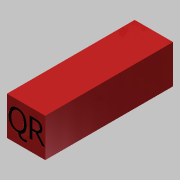
# Autodesk Inventor part: Container 2 2 5 colored color 4
Saved by Autodesk Inventor 2015 (Build 190159000, 159)
## iProperties
Created: 2015-03-07
Part Number: Container 2 2 5 colored color 4
Material: Generic
Document SubType Name: Modeling
Designer: Vukica
Density: 1 g/cm^3
Appearance: Light Red
Author: Vukica
Autodesk Inventor part; units mm, degrees
ref_plane "YZ Plane" through (0, 0, 0) normal (1, 0, 0) x (0, 1, 0)
ref_plane "XZ Plane" through (0, 0, 0) normal (0, 1, 0) x (-1, 0, 0)
ref_plane "XY Plane" through (0, 0, 0) normal (0, 0, 1) x (1, 0, 0)
sketch "Sketch1" plane through (0, 0, 0) normal (0, 0, 1) x (1, 0, 0)
  line L0 (0, 0) -> (38.1, 0)
  line L1 (38.1, 0) -> (38.1, 38.1)
  line L2 (38.1, 38.1) -> (0, 38.1)
  line L3 (0, 38.1) -> (0, 0)
  dimension "d0" = 38.1
  dimension "d1" = 38.1
  constraints: 8 end point, 2 parallel, 1 horizontal, 1 perpendicular
  measures "d0" distance of L1.end L2.end
  measures "d1" distance of L2.end L0.start
extrude "Extrusion1" add sketch "Sketch1" along normal blind 127
sketch "Sketch2" plane through (0, 0, 127) normal (0, 0, 1) x (1, 0, 0)
  line L0 (0.6292, 31.1418) -> (47.0243, 31.1418) construction
  line L1 (47.0243, 31.1418) -> (47.0243, -1.483) construction
  line L2 (47.0243, -1.483) -> (0.6292, -1.483) construction
  line L3 (0.6292, -1.483) -> (0.6292, 31.1418) construction
  spline S0 degree 2 poles (19.566, 5.4207) (18.825, 5.2396) (17.2112, 5.042) (16.4044, 5.042) knots 0 0 0 1 2 2 2
  spline S1 degree 2 poles (16.4044, 5.042) (14.1155, 5.042) (11.2667, 7.5944) (11.135, 9.9656) knots 0 0 0 1 2 2 2
  spline S2 degree 2 poles (11.135, 9.9656) (10.9539, 9.9656) (10.641, 9.9656) (10.5093, 9.9656) knots 0 0 0 1 2 2 2
  spline S3 degree 2 poles (10.5093, 9.9656) (8.4509, 9.9656) (5.1411, 11.3652) (3.9555, 12.732) knots 0 0 0 1 2 2 2
  spline S4 degree 2 poles (3.9555, 12.732) (2.7863, 14.0823) (1.5349, 18.0343) (1.5349, 20.5372) knots 0 0 0 1 2 2 2
  spline S5 degree 2 poles (1.5349, 20.5372) (1.5349, 23.1061) (2.8028, 26.9922) (3.972, 28.3754) knots 0 0 0 1 2 2 2
  spline S6 degree 2 poles (3.972, 28.3754) (5.1576, 29.7422) (8.4674, 31.1418) (10.5093, 31.1418) knots 0 0 0 1 2 2 2
  spline S7 degree 2 poles (10.5093, 31.1418) (12.5841, 31.1418) (15.9104, 29.6928) (17.063, 28.3754) knots 0 0 0 1 2 2 2
  spline S8 degree 2 poles (17.063, 28.3754) (18.2157, 27.0416) (19.5001, 23.0731) (19.5001, 20.5372) knots 0 0 0 1 2 2 2
  spline S9 degree 2 poles (19.5001, 20.5372) (19.5001, 16.5852) (16.4208, 11.4476) (13.7368, 10.5419) knots 0 0 0 1 2 2 2
  spline S10 degree 2 poles (13.7368, 10.5419) (13.8026, 9.7844) (14.1978, 8.5659) (14.5107, 8.2201) knots 0 0 0 1 2 2 2
  spline S11 degree 2 poles (14.5107, 8.2201) (14.8894, 7.792) (15.9268, 7.3968) (16.849, 7.3968) knots 0 0 0 1 2 2 2
  spline S12 degree 2 poles (16.849, 7.3968) (17.3924, 7.3968) (18.8744, 7.7426) (19.2037, 7.8743) knots 0 0 0 1 2 2 2
  line L4 (19.2037, 7.8743) -> (19.566, 7.8743)
  line L5 (19.566, 7.8743) -> (19.566, 5.4207)
  spline S13 degree 2 poles (16.6843, 20.5372) (16.6843, 22.5627) (15.8116, 25.6749) (15.0212, 26.6958) knots 0 0 0 1 2 2 2
  spline S14 degree 2 poles (15.0212, 26.6958) (14.2143, 27.7497) (11.9419, 28.8036) (10.5257, 28.8036) knots 0 0 0 1 2 2 2
  spline S15 degree 2 poles (10.5257, 28.8036) (9.0602, 28.8036) (6.8536, 27.7826) (6.0138, 26.6958) knots 0 0 0 1 2 2 2
  spline S16 degree 2 poles (6.0138, 26.6958) (5.207, 25.6584) (4.3507, 22.5133) (4.3507, 20.5372) knots 0 0 0 1 2 2 2
  spline S17 degree 2 poles (4.3507, 20.5372) (4.3507, 16.5358) (7.7099, 12.2709) (10.5257, 12.2709) knots 0 0 0 1 2 2 2
  spline S18 degree 2 poles (10.5257, 12.2709) (13.3416, 12.2709) (16.6843, 16.5358) (16.6843, 20.5372) knots 0 0 0 1 2 2 2
  line L6 (38.1899, 10.3937) -> (34.6825, 10.3937)
  line L7 (34.6825, 10.3937) -> (28.2605, 18.4789)
  line L8 (28.2605, 18.4789) -> (25.1647, 18.4789)
  line L9 (25.1647, 18.4789) -> (25.1647, 10.3937)
  line L10 (25.1647, 10.3937) -> (22.4641, 10.3937)
  line L11 (22.4641, 10.3937) -> (22.4641, 30.7137)
  line L12 (22.4641, 30.7137) -> (27.7006, 30.7137)
  spline S19 degree 2 poles (27.7006, 30.7137) (29.4461, 30.7137) (31.8008, 30.335) (32.8711, 29.6434) knots 0 0 0 1 2 2 2
  spline S20 degree 2 poles (32.8711, 29.6434) (33.9415, 28.9518) (35.1765, 26.7946) (35.1765, 25.1973) knots 0 0 0 1 2 2 2
  spline S21 degree 2 poles (35.1765, 25.1973) (35.1765, 22.9743) (32.9041, 19.9609) (30.961, 19.2364) knots 0 0 0 1 2 2 2
  line L13 (30.961, 19.2364) -> (38.1899, 10.3937)
  spline S22 degree 2 poles (32.3607, 24.9833) (32.3607, 25.8725) (31.7349, 27.2392) (31.0763, 27.6838) knots 0 0 0 1 2 2 2
  spline S23 degree 2 poles (31.0763, 27.6838) (30.4999, 28.0626) (28.9685, 28.3754) (27.8488, 28.3754) knots 0 0 0 1 2 2 2
  line L14 (27.8488, 28.3754) -> (25.1647, 28.3754)
  line L15 (25.1647, 28.3754) -> (25.1647, 20.7348)
  line L16 (25.1647, 20.7348) -> (27.5359, 20.7348)
  spline S24 degree 2 poles (27.5359, 20.7348) (28.7051, 20.7348) (30.5658, 21.1465) (31.208, 21.7887) knots 0 0 0 1 2 2 2
  spline S25 degree 2 poles (31.208, 21.7887) (31.8008, 22.3486) (32.3607, 23.9294) (32.3607, 24.9833) knots 0 0 0 1 2 2 2
  point P0 (0, 0)
  constraints: 2 other
extrude "Extrusion3" cut sketch "Sketch2" against normal blind 0.254
body "Solid1"
